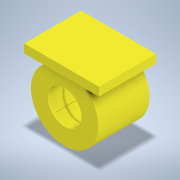
# Autodesk Inventor part: Part8
Saved by Autodesk Inventor 2020 (Build 240168000, 168)
## iProperties
Created: 2022-04-26
Part Number: Part8
Material: Steel
Document SubType Name: Modeling
Designer: Manish
Density: 7.85 g/cm^3
Appearance: Plate
Mass: 4330.19 g
Surface Area: 656.393 cm^2
Volume: 551.616 cm^3
Author: Manish
Autodesk Inventor part; units mm, degrees
ref_plane "YZ Plane" through (0, 0, 0) normal (1, 0, 0) x (0, 1, 0)
ref_plane "XY Plane" through (0, 0, 0) normal (0, 0, 1) x (1, 0, 0)
sketch "Sketch1" plane through (0, 0, 0) normal (0, 0, 1) x (1, 0, 0)
  circle A0 centre (0, 0) radius 50
  circle A1 centre (0, 0) radius 25
  dimension "d0" = 100
  dimension "d1" = 50
  constraints: 2 centre point, 2 coincident
  measures "d0" diameter of A0
  measures "d1" diameter of A1
extrude "Extrusion1" add sketch "Sketch1" along normal blind 76.2
ref_plane "Work Plane1" through (0, 50, 0) normal (0, 1, 0) x (-1, 0, 0)
sketch "Sketch2" plane through (0, 50, 0) normal (0, 1, 0) x (-1, 0, 0)
  line L0 (55.6155, 80.6654) -> (-55.6155, 80.6654)
  line L1 (-55.6155, 80.6654) -> (-55.6155, -3.9069)
  line L2 (-55.6155, -3.9069) -> (55.6155, -3.9069)
  line L3 (55.6155, -3.9069) -> (55.6155, 80.6654)
  point P0 (0, 0)
  constraints: 8 end point, 2 parallel, 1 horizontal, 1 perpendicular
extrude "Extrusion2" add sketch "Sketch2" along normal mid plane 12.7
sketch "Sketch3" plane through (0, 0, 76.2) normal (0, 0, 1) x (1, 0, 0)
  circle A0 centre (0, 0) radius 25 projected
  circle A1 centre (-21.939, 11.9866) radius 2.5
  dimension "d7" = 5
  constraints: 1 centre point, 2 other
  measures "d7" diameter of A1
coil "Coil1" sketch "Sketch3" operation cut axis through (0, 0, 0) along (0, 0, -1) pitch 25.4 turns 3 hand right contours A1 A0 | A0 A1
body "Solid1"
